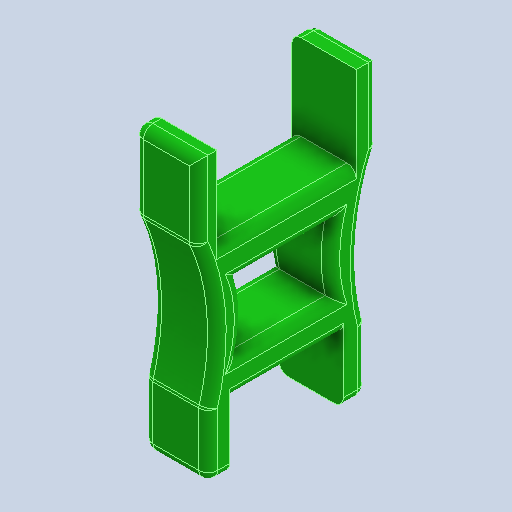
# Autodesk Inventor part: arm_mid_link2
Saved by Autodesk Inventor 2022 (Build 260153000, 153)
## iProperties
Created: 2022-04-25
Part Number: arm_mid_link2
Material: Generic
Document SubType Name: Modeling
Designer: HP
Density: 1 g/cm^3
Appearance: Dark Green
Author: HP
Autodesk Inventor part; units mm, degrees
ref_plane "YZ Plane" through (0, 0, 0) normal (1, 0, 0) x (0, 1, 0)
ref_plane "XZ Plane" through (0, 0, 0) normal (0, 1, 0) x (-1, 0, 0)
ref_plane "XY Plane" through (0, 0, 0) normal (0, 0, 1) x (1, 0, 0)
sketch "Sketch2" plane through (0, 0, 0) normal (1, 0, 0) x (0, 1, 0)
  line L0 (-11.003, -19.3563) -> (11.003, -19.3563)
  line L1 (11.003, -19.3563) -> (11.003, 19.3563)
  line L2 (11.003, 19.3563) -> (-11.003, 19.3563)
  line L3 (57.7702, -23.7983) -> (86.9201, -23.7983)
  line L4 (86.9201, 23.7983) -> (57.7702, 23.7983)
  line L5 (57.7702, 23.7983) -> (57.7702, -23.7983)
  line L6 (57.7702, -23.7983) -> (60.4906, -19.3563) construction
  line L7 (60.4906, 19.3563) -> (57.7702, 23.7983) construction
  line L8 (86.9201, 29.9796) -> (60.767, 29.9796)
  line L9 (86.9201, -31.153) -> (60.767, -31.153)
  line L10 (-11.003, -27.448) -> (11.003, -27.448)
  line L11 (-11.003, 26.7377) -> (11.003, 26.7377)
  arc A0 (11.003, 26.7377) -> (60.767, 29.9796) centre (31.4829, 95.932) ccw
  arc A1 (60.767, -31.153) -> (11.003, -27.448) centre (30.5123, -101.4643) ccw
  line L12 (45.6284, 16.3623) -> (45.6284, -16.3623)
  line L13 (22.3276, 16.3623) -> (22.3276, -16.3623)
  arc A2 (22.3276, 16.3623) -> (45.6284, 16.3623) centre (33.978, 54.9478) ccw
  arc A3 (45.6284, -16.3623) -> (22.3276, -16.3623) centre (33.978, -64.7297) ccw
  line L14 (-11.003, 26.7377) -> (-11.003, 19.3563)
  line L15 (-11.003, -19.3563) -> (-11.003, -27.448)
  line L16 (86.9201, 29.9796) -> (86.9201, 23.7983)
  line L17 (86.9201, -23.7983) -> (86.9201, -31.153)
  point P0 (0, 0)
  constraints: 36 end point, 8 point on circle, 6 horizontal, 4 centre point, 4 vertical, 2 collinear, 2 parallel, 2 point on line, 1 perpendicular
extrude "Extrusion2" add sketch "Sketch2" along normal blind 22
fillet "Fillet2" radius 3.175 38 edges at (22, 73.8435, 29.9796) (11, 60.767, 29.9796) (0, 73.8435, 29.9796) (0, 36.1739, 23.9231) (22, 36.1739, 23.9231) (22, 57.7702, 0) (22, 45.6284, 0) (22, 22.3276, 0) (22, 11.003, 0) (22, 33.978, -14.9789) (22, 33.978, 14.6418) (22, 36.1954, -25.1313) (22, 73.8435, -31.153) (11, 86.9201, -31.153) (11, 86.9201, 29.9796) (11, 11.003, 26.7377) (22, 0, 26.7377) (0, 0, 26.7377) (22, 0, -27.448) (0, 73.8435, -31.153) (11, 60.767, -31.153) (0, 36.1954, -25.1313) (11, 11.003, -27.448) (0, 22.3276, 0) (0, 45.6284, 0) (0, 33.978, 14.6418) (0, 33.978, -14.9789) (0, 0, -27.448) (11, -11.003, -27.448) (11, -11.003, 26.7377) (0, 11.003, 0) (0, 57.7702, 0) (0, 86.9201, -27.4756) (0, 86.9201, 26.889) (0, -11.003, -23.4021) (0, -11.003, 23.047) (22, -11.003, 23.047) (22, -11.003, -23.4021)
body "Solid2"
